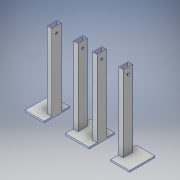
# Autodesk Inventor part: RearPostForLiftV02
Saved by Autodesk Inventor 2016 SP1 (Build 200210100, 210)
## iProperties
Created: 2016-02-01
Part Number: RearPostForLiftV02
Material: Aluminum 6061
Document SubType Name: Modeling
Designer: steele
Density: 2.7 g/cm^3
Appearance: Aluminum - Flat
Mass: 1488.38 g
Surface Area: 3047 cm^2
Volume: 551.254 cm^3
Author: steele
Autodesk Inventor part; units mm, degrees
ref_plane "YZ Plane" through (0, 0, 0) normal (1, 0, 0) x (0, 1, 0)
ref_plane "XZ Plane" through (0, 0, 0) normal (0, 1, 0) x (-1, 0, 0)
ref_plane "XY Plane" through (0, 0, 0) normal (0, 0, 1) x (1, 0, 0)
sketch "Sketch1" plane through (0, 0, 0) normal (0, 1, 0) x (-1, 0, 0)
  line L0 (47.625, 50.8) -> (-47.625, 50.8)
  line L1 (-47.625, 50.8) -> (-47.625, -50.8)
  line L2 (-47.625, -50.8) -> (47.625, -50.8)
  line L3 (47.625, -50.8) -> (47.625, 50.8)
  line L4 (47.625, 50.8) -> (-47.625, -50.8) construction
  line L5 (-47.625, 50.8) -> (47.625, -50.8) construction
  point P0 (0, 0)
  dimension "d0" = 95.25
  dimension "d1" = 101.6
  constraints: 12 end point, 2 midpoint, 2 parallel, 1 horizontal, 1 perpendicular
  measures "d0" distance of L0.start L0.end
  measures "d1" distance of L2.end L0.start
extrude "Extrusion1" add sketch "Sketch1" against normal blind 6.35
sketch "Sketch2" plane through (0, 0, 0) normal (0, 1, 0) x (1, 0, 0)
  line L0 (-47.625, -19.05) -> (-28.575, -19.05)
  line L1 (-28.575, -19.05) -> (-28.575, 19.05)
  line L2 (-28.575, 19.05) -> (-47.625, 19.05)
  line L3 (-47.625, 19.05) -> (-47.625, -19.05)
  line L4 (-47.625, -19.05) -> (-28.575, 19.05) construction
  line L5 (-28.575, -19.05) -> (-47.625, 19.05) construction
  line L6 (-44.45, -15.875) -> (-31.75, -15.875)
  line L7 (-31.75, -15.875) -> (-31.75, 15.875)
  line L8 (-31.75, 15.875) -> (-44.45, 15.875)
  line L9 (-44.45, 15.875) -> (-44.45, -15.875)
  line L10 (-44.45, -15.875) -> (-31.75, 15.875) construction
  line L11 (-31.75, -15.875) -> (-44.45, 15.875) construction
  line L12 (-47.625, 50.8) -> (47.625, 50.8) construction
  line L13 (0, 50.8) -> (0, -101.6) construction
  line L14 (47.625, -19.05) -> (28.575, -19.05)
  line L15 (28.575, -19.05) -> (28.575, 19.05)
  line L16 (28.575, 19.05) -> (47.625, 19.05)
  line L17 (47.625, 19.05) -> (47.625, -19.05)
  line L18 (44.45, -15.875) -> (31.75, -15.875)
  line L19 (31.75, -15.875) -> (31.75, 15.875)
  line L20 (31.75, 15.875) -> (44.45, 15.875)
  line L21 (44.45, 15.875) -> (44.45, -15.875)
  point P0 (0, 0)
  point P1 (-38.1, 0)
  dimension "d4" = 38.1
  dimension "d5" = 19.05
  dimension "d6" = 38.1
  dimension "d7" = 3.175
  dimension "d8" = 3.175
  constraints: 42 end point, 8 symmetric about line, 5 midpoint, 4 parallel, 2 horizontal, 2 perpendicular, 1 vertical
  measures "d4" distance of point (0, 0) point (-38.1, 0)
  measures "d5" distance of L0.start L0.end
  measures "d6" distance of L2.end L0.start
  measures "d7" distance between parallel lines of L0 L6
  measures "d8" distance between parallel lines of L9 L3
extrude "Extrusion2" add sketch "Sketch2" along normal blind 304.8
sketch "Sketch4" plane through (-47.625, -6.35, -50.8) normal (-1, 0, 0) x (0, 0, 1)
  line L0 (50.8, 6.35) -> (50.8, 96.458) construction
  circle A0 centre (50.8, 285.75) radius 4.7625
  line L1 (0, 6.35) -> (31.75, 6.35) projected
  dimension "d15" = 9.525
  dimension "d16" = 279.4
  constraints: 2 end point, 1 centre point, 1 point on line, 1 vertical
  measures "d15" diameter of A0
  measures "d16" distance from line of A0.centre L1
extrude "Extrusion4" cut sketch "Sketch4" against normal through all
sketch "Sketch6" plane through (0, 0, 0) normal (0, 1, 0) x (-1, 0, 0)
  line L0 (209.55, 50.8) -> (133.35, 50.8)
  line L1 (133.35, 50.8) -> (133.35, -50.8)
  line L2 (133.35, -50.8) -> (209.55, -50.8)
  line L3 (209.55, -50.8) -> (209.55, 50.8)
  line L4 (209.55, 50.8) -> (133.35, -50.8) construction
  line L5 (133.35, 50.8) -> (209.55, -50.8) construction
  point P0 (0, 0)
  point P1 (171.45, 0)
  dimension "d19" = 101.6
  dimension "d20" = 76.2
  dimension "d21" = 209.55
  constraints: 12 end point, 2 midpoint, 2 parallel, 1 horizontal, 1 perpendicular
  measures "d19" distance of L2.end L0.start
  measures "d20" distance of L0.start L0.end
  measures "d21" distance from line of point (0, 0) L3
extrude "Extrusion5" add sketch "Sketch6" against normal blind 6.35
sketch "Sketch7" plane through (0, 0, 0) normal (0, 1, 0) x (1, 0, 0)
  line L0 (-152.4, -19.1787) -> (-133.35, -19.1787)
  line L1 (-133.35, -19.1787) -> (-133.35, 18.9213)
  line L2 (-133.35, 18.9213) -> (-152.4, 18.9213)
  line L3 (-152.4, 18.9213) -> (-152.4, -19.1787)
  line L4 (-152.4, -19.1787) -> (-133.35, 18.9213) construction
  line L5 (-133.35, -19.1787) -> (-152.4, 18.9213) construction
  line L6 (-149.225, -16.0037) -> (-136.525, -16.0037)
  line L7 (-136.525, -16.0037) -> (-136.525, 15.7463)
  line L8 (-136.525, 15.7463) -> (-149.225, 15.7463)
  line L9 (-149.225, 15.7463) -> (-149.225, -16.0037)
  line L10 (-149.225, -16.0037) -> (-136.525, 15.7463) construction
  line L11 (-136.525, -16.0037) -> (-149.225, 15.7463) construction
  line L12 (-133.35, -50.8) -> (-133.35, 50.8) projected
  point P0 (0, 0)
  point P1 (-142.875, -0.1287)
  dimension "d24" = 19.05
  dimension "d25" = 38.1
  dimension "d26" = 3.175
  dimension "d27" = 3.175
  constraints: 24 end point, 4 midpoint, 4 parallel, 2 horizontal, 2 perpendicular, 1 collinear
  measures "d24" distance of L0.start L0.end
  measures "d25" distance of L2.end L0.start
  measures "d26" distance between parallel lines of L6 L0
  measures "d27" distance between parallel lines of L3 L9
extrude "Extrusion6" add sketch "Sketch7" along normal blind 304.8
sketch "Sketch8" plane through (-133.35, -6.35, 50.8) normal (1, 0, 0) x (0, 0, -1)
  line L0 (50.8, 6.35) -> (50.6713, 311.15) construction
  line L1 (34.7963, 311.15) -> (66.5463, 311.15) construction
  circle A0 centre (50.682, 285.75) radius 4.7625
  line L2 (101.6, 6.35) -> (0, 6.35) projected
  dimension "d30" = 9.525
  dimension "d31" = 279.4
  constraints: 2 end point, 1 centre point, 1 midpoint, 1 point on line
  measures "d30" diameter of A0
  measures "d31" distance from line of A0.centre L2
extrude "Extrusion7" cut sketch "Sketch8" against normal through all
mirror "Mirror1" about plane through (0, 0, 0) normal (1, 0, 0) of "Extrusion6", "Extrusion7", "Extrusion5"
equation "\"d0\" = BaseWidth"
equation "\"d1\" = BaseLength"
equation "\"d2\" = BaseThickness"
equation "\"d4\" = postCenterDistanceFromCenterOfBase"
equation "\"d5\" = postWidth"
equation "\"d6\" = postLength"
equation "\"d7\" = postThickness"
equation "\"d8\" = postThickness"
equation "\"d9\" = postHeight"
equation "\"d15\" = axelDiam"
equation "\"d16\" = axelHeightAbovePlate"
equation "\"d19\" = BaseLength"
equation "\"d20\" = baseForArmWidth"
equation "\"d21\" = 0.5 * robotBaseWidth"
equation "\"d22\" = BaseThickness"
equation "\"d24\" = postWidth"
equation "\"d25\" = postLength"
equation "\"d26\" = postThickness"
equation "\"d27\" = postThickness"
equation "\"d28\" = postHeight"
equation "\"d30\" = axelDiam"
equation "\"d31\" = axelHeightAbovePlate"
equation "\"d32\" = postHeight"
equation "\"BaseWidth\" = 95.25"
equation "\"BaseLength\" = 101.6"
equation "\"BaseThickness\" = 6.35"
equation "\"postWidth\" = 19.05"
equation "\"postLength\" = 38.1"
equation "\"postThickness\" = 3.175"
equation "\"postCenterDistanceFromCenterOfBase\" = 38.1"
equation "\"postHeight\" = 304.8"
equation "\"axelDiam\" = 9.525"
equation "\"baseForArmWidth\" = 76.2"
equation "\"robotBaseWidth\" = 419.1"
equation "\"telescopeArmWidth\" = 44.45"
equation "\"postToSupportArmAxelDistanceFromCenter\" = 0.5 * robotBaseWidth - baseForArmWidth"
equation "\"axelHeightAbovePlate\" = 279.4"
body "Solid1"
